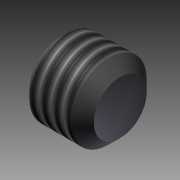
# Autodesk Inventor part: SET-SCREW5-4
Saved by Autodesk Inventor 2011 SP1 (Build 150282100, 282)
## iProperties
Created: 2016-11-23
Part Number: SET-SCREW5-4
Catalog Web Link: www.cadenas.de
Description: SET-SCREW-Set Screw - Flat End
Vendor: MISUMI
Document SubType Name: Modeling
Designer: psAdmin
Manufacturer: MISUMI
Mass: 0.0607915 g
Surface Area: 1.07722 cm^2
Volume: 0.0607915 cm^3
Density: 1 g/cm^3
Category: PARTsolutions
Company: MISUMI
Title: SET-SCREW5-4
Author: Cadenas PARTsolutions
Comments: Set Screw - Flat End
PSOL_IDENT_0: {$CADENAS_DATA\23d-libs\misumi\metric\accessories\set_screw.prj},170 {VTYP=3D},{NB=SET-SCREW5-4},{LI
PSOL_IDENT_1: NA=SET-SCREW5-4},{NN=SET-SCREW},{DATE=17.06.2016 05:56:50},{GEOMDATE=11.12.2013 00:00:00},{VERSION=}
PSOL_IDENT_2: ,{LINEID=80},{LINESUBID=-1},{WBVAR=L}  {NB=SET-SCREW5-4},{LINA=SET-SCREW5-4},{KT=DUMMY},{PN=SET-SCRE
PSOL_IDENT_3: W5-4},{TYPE=SET-SCREW},{M=5.0},{P=0.80},{L=4},{LMIN=2.8},{LALG=[2.8:42/0.1]},{B=2.5},{C=2.0},{DD=3.5
PSOL_IDENT_4: }
NN: SET-SCREW
NT: Set Screw - Flat End
NB: SET-SCREW5-4
NBSYN: $PN.
LINA: SET-SCREW5-4
PN: SET-SCREW5-4
M: 5.0
P: 0.80
L: 4.0
B: 2.5
C: 2.0
DD: 3.5
SUPPLIER: MISUMI
ARTICLENO: SET-SCREW5-4
BOMINFO: SET-SCREW5-4
CREATOR: CADENAS GmbH
Autodesk Inventor part; units mm, degrees
sketch "Sketch_1" plane through (0, 0, 0) normal (0, 0, 1) x (1, 0, 0)
  line L0 (0, 0) -> (-4, 0)
  line L1 (-4, 0) -> (-4, 2.0095)
  line L2 (-4, 2.0095) -> (-3.5095, 2.5)
  line L3 (-3.5095, 2.5) -> (-0.75, 2.5)
  line L4 (-0.75, 2.5) -> (0, 1.75)
  line L5 (0, 1.75) -> (0, 0)
  line L6 (0, 0) -> (-4, 0)
  constraints: 14 end point
revolve "Revolution1" add sketch "Sketch_1" angle 360 about axis through (0, 0, 0) along (1, 0, 0)
thread "Thread1" size "M5x0.8" class "6g" standard "ISO Metric profile" full length
sketch "Sketch_2" plane through (-4, 0, 0) normal (-1, 0, 0) x (0, 1, 0)
  line L0 (-1.25, 0.7217) -> (-1.25, -0.7217)
  line L1 (-1.25, -0.7217) -> (0, -1.4434)
  line L2 (0, -1.4434) -> (1.25, -0.7217)
  line L3 (1.25, -0.7217) -> (1.25, 0.7217)
  line L4 (1.25, 0.7217) -> (0, 1.4434)
  line L5 (0, 1.4434) -> (-1.25, 0.7217)
  constraints: 12 end point
extrude "Extrusion1" cut sketch "Sketch_2" against normal blind 2
sketch "Sketch_3" plane through (0, 0, 0) normal (0, 0, 1) x (1, 0, 0)
  line L0 (-1.2783, 0) -> (-2, 0)
  line L1 (-2, 0) -> (-2, 1.25)
  line L2 (-2, 1.25) -> (-1.2783, 0)
  line L3 (-1.2783, 0) -> (-2, 0)
  constraints: 8 end point
revolve "Revolution2" cut sketch "Sketch_3" angle 360 about axis through (-1.2783, 0, 0) along (1, 0, 0)
ref_plane "CP_XY" through (0, 0, 0) normal (1, 0, 0) x (0, 0, -1)
ref_plane "CP_YZ" through (0, 0, 0) normal (0, 0, -1) x (0, 1, 0)
ref_plane "CP_ZX" through (0, 0, 0) normal (0, 1, 0) x (1, 0, 0)
body "Solid1"
